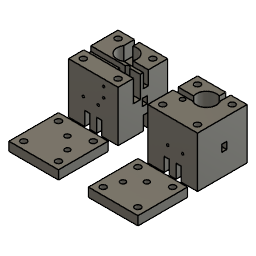
midrail support (Autodesk Fusion 360 design; units mm, degrees)
Autodesk Fusion 360 part; units mm, degrees
note: some values were not read from the file. Chosen so that the rebuilt part matches the saved one: which face or edge a step refers to. Set by a fixed rule: which sketch regions a step uses.
sketch "Sketch1" plane through (0, 0, 0) normal (0, 1, 0) x (1, 0, 0)
  line L0 (25, -25) -> (-25, -25)
  line L1 (-25, -25) -> (-25, 25)
  line L2 (-25, 25) -> (25, 25)
  line L3 (25, 25) -> (25, -25)
  line L4 (25, -25) -> (-25, 25) construction
  line L5 (-25, -25) -> (25, 25) construction
  line L6 (17.5, -17.5) -> (-17.5, -17.5)
  line L7 (-17.5, -17.5) -> (-17.5, 17.5)
  line L8 (-17.5, 17.5) -> (17.5, 17.5)
  line L9 (17.5, 17.5) -> (17.5, -17.5)
  line L10 (17.5, -17.5) -> (-17.5, 17.5) construction
  line L11 (-17.5, -17.5) -> (17.5, 17.5) construction
  circle A0 centre (-17.5, 17.5) radius 1.95
  circle A1 centre (17.5, 17.5) radius 1.95
  circle A2 centre (17.5, -17.5) radius 1.95
  circle A3 centre (-17.5, -17.5) radius 1.95
  line L12 (25, 0) -> (25, 3.5)
  line L13 (-25, 3.5) -> (-25, 0)
  line L14 (25, 0) -> (25, -1.5)
  circle A4 centre (-17.5, 17.5) radius 3
  circle A5 centre (17.5, 17.5) radius 3
  circle A6 centre (17.5, -17.5) radius 3
  circle A7 centre (-17.5, -17.5) radius 3
  line L15 (-25, 2.5) -> (-25, -2.5)
  line L16 (25, -2.5) -> (25, 2.5)
  line L17 (25, 2.5) -> (-25, -2.5) construction
  line L18 (-25, 2.5) -> (25, -2.5) construction
  line L19 (-14.5, -17.5) -> (-13, -17.5)
  line L20 (-13, 17.5) -> (-14.5, 17.5)
  line L21 (-13, -17.5) -> (-8, -17.5)
  line L22 (-8, -25) -> (-13, -25)
  line L23 (-8, -25) -> (-13, -25)
  line L24 (-13, 25) -> (-8, 25)
  line L25 (-10.5, 25) -> (1.5, 25)
  line L26 (1.5, -25) -> (-10.5, -25)
  line L27 (1.5, -25) -> (-1, -25)
  line L28 (1.5, -25) -> (4, -25)
  line L29 (6, -25) -> (-6, -25)
  line L30 (-6, -25) -> (-6, 25)
  line L31 (-6, 25) -> (6, 25)
  line L32 (6, 25) -> (6, -25)
  line L33 (6, -25) -> (-6, 25) construction
  line L34 (-6, -25) -> (6, 25) construction
  line L35 (8.5, -25) -> (3.5, -25)
  line L36 (3.5, -25) -> (3.5, 25)
  line L37 (3.5, 25) -> (8.5, 25)
  line L38 (8.5, 25) -> (8.5, -25)
  line L39 (8.5, -25) -> (3.5, 25) construction
  line L40 (3.5, -25) -> (8.5, 25) construction
  line L41 (-3.5, -25) -> (-8.5, -25)
  line L42 (-8.5, -25) -> (-8.5, 25)
  line L43 (-8.5, 25) -> (-3.5, 25)
  line L44 (-3.5, 25) -> (-3.5, -25)
  line L45 (-3.5, -25) -> (-8.5, 25) construction
  line L46 (-8.5, -25) -> (-3.5, 25) construction
  line L47 (25, 0) -> (-25, 0)
  line L48 (-25, 0) -> (-25, 3)
  line L49 (-25, 3) -> (25, 3)
  line L50 (25, 3) -> (25, 0)
  line L51 (25, 0.5) -> (-25, 0.5)
  line L52 (-25, 0.5) -> (-25, 5.5)
  line L53 (-25, 5.5) -> (25, 5.5)
  line L54 (25, 5.5) -> (25, 0.5)
  line L55 (25, 0.5) -> (-25, 5.5) construction
  line L56 (-25, 0.5) -> (25, 5.5) construction
  line L57 (6, 3) -> (12, 3)
  line L58 (12, 3) -> (12, -3)
  line L59 (12, -3) -> (6, -3)
  line L60 (6, -3) -> (6, 3)
  circle A8 centre (12, -3) radius 10
  line L61 (-6, 3) -> (0, 3)
  line L62 (0, 3) -> (0, 9)
  line L63 (0, 9) -> (-6, 9)
  line L64 (-6, 9) -> (-6, 3)
  circle A9 centre (0, 9) radius 10
  circle A10 centre (12, -3) radius 2.4
  circle A11 centre (0, 9) radius 2.4
  line L65 (25, 3) -> (-25, 3)
  line L66 (-25, 3) -> (-25, -0.5)
  line L67 (-25, -0.5) -> (25, -0.5)
  line L68 (25, -0.5) -> (25, 3)
  line L69 (25, 3) -> (-25, 3)
  line L70 (-25, 3) -> (-25, 4.5)
  line L71 (-25, 4.5) -> (25, 4.5)
  line L72 (25, 4.5) -> (25, 3)
  line L73 (25, -57) -> (-25, -57)
  line L74 (-25, -85) -> (-25, -35)
  line L75 (6, -57) -> (12, -57)
  line L76 (12, -63) -> (6, -63)
  line L77 (-6, -85) -> (-6, -35)
  line L78 (-8.5, -85) -> (-8.5, -35)
  line L79 (17.5, -42.5) -> (17.5, -77.5)
  line L80 (-25, -59.5) -> (-25, -54.5)
  line L81 (1.5, -85) -> (4, -85)
  circle A12 centre (-17.5, -77.5) radius 2.1
  line L82 (-25, -57.5) -> (-25, -62.5)
  line L83 (-25, -60) -> (-25, -57)
  circle A13 centre (17.5, -42.5) radius 2.1
  circle A14 centre (17.5, -77.5) radius 3
  line L84 (-8.5, -85) -> (-3.5, -35) construction
  line L85 (-3.5, -85) -> (-8.5, -35) construction
  line L86 (-25, -57) -> (-25, -55.5)
  line L87 (25, -57) -> (-25, -57)
  line L88 (-17.5, -77.5) -> (17.5, -42.5) construction
  line L89 (-25, -85) -> (25, -35) construction
  circle A15 centre (12, -63) radius 10
  line L90 (-25, -56.5) -> (-25, -60)
  line L91 (-6, -35) -> (6, -35)
  line L92 (6, -85) -> (-6, -35) construction
  circle A16 centre (0, -51) radius 10
  line L93 (25, -60) -> (-25, -60)
  line L94 (25, -59.5) -> (-25, -54.5) construction
  line L95 (-25, -60.5) -> (25, -60.5)
  line L96 (17.5, -77.5) -> (-17.5, -42.5) construction
  line L97 (17.5, -77.5) -> (-17.5, -77.5)
  line L98 (-25, -57) -> (-25, -60.5)
  line L99 (6, -85) -> (-6, -85)
  line L100 (-6, -85) -> (6, -35) construction
  line L101 (-6, -57) -> (0, -57)
  line L102 (-17.5, -77.5) -> (-17.5, -42.5)
  line L103 (-13, -77.5) -> (-8, -77.5)
  line L104 (25, -60.5) -> (25, -57)
  circle A17 centre (17.5, -77.5) radius 2.1
  line L105 (8.5, -35) -> (8.5, -85)
  line L106 (-8, -85) -> (-13, -85)
  line L107 (25, -54.5) -> (25, -59.5)
  line L108 (3.5, -85) -> (8.5, -35) construction
  line L109 (-3.5, -35) -> (-3.5, -85)
  line L110 (1.5, -85) -> (-10.5, -85)
  circle A18 centre (-17.5, -42.5) radius 2.1
  line L111 (25, -57) -> (25, -60)
  line L112 (3.5, -35) -> (8.5, -35)
  line L113 (0, -51) -> (-6, -51)
  line L114 (1.5, -85) -> (-1, -85)
  line L115 (-13, -42.5) -> (-14.5, -42.5)
  line L116 (-3.5, -85) -> (-8.5, -85)
  line L117 (-25, -55.5) -> (25, -55.5)
  line L118 (-17.5, -42.5) -> (17.5, -42.5)
  line L119 (25, -59.5) -> (-25, -59.5)
  line L120 (-25, -35) -> (25, -35)
  line L121 (-25, -57) -> (25, -57)
  line L122 (25, -85) -> (-25, -85)
  line L123 (-25, -59.5) -> (25, -54.5) construction
  circle A19 centre (-17.5, -77.5) radius 3
  circle A20 centre (-17.5, -42.5) radius 3
  line L124 (-25, -54.5) -> (25, -54.5)
  line L125 (25, -57.5) -> (-25, -62.5) construction
  circle A21 centre (12, -63) radius 2.6
  line L126 (6, -63) -> (6, -57)
  line L127 (-6, -51) -> (-6, -57)
  line L128 (-8, -85) -> (-13, -85)
  line L129 (0, -57) -> (0, -51)
  line L130 (-14.5, -77.5) -> (-13, -77.5)
  line L131 (-13, -35) -> (-8, -35)
  line L132 (-10.5, -35) -> (1.5, -35)
  line L133 (8.5, -85) -> (3.5, -35) construction
  circle A22 centre (17.5, -42.5) radius 3
  line L134 (25, -60) -> (25, -56.5)
  line L135 (25, -35) -> (25, -85)
  line L136 (25, -55.5) -> (25, -57)
  line L137 (-8.5, -35) -> (-3.5, -35)
  line L138 (3.5, -85) -> (3.5, -35)
  line L139 (12, -57) -> (12, -63)
  line L140 (25, -62.5) -> (25, -57.5)
  line L141 (6, -35) -> (6, -85)
  line L142 (8.5, -85) -> (3.5, -85)
  line L143 (25, -60) -> (25, -61.5)
  line L144 (25, -85) -> (-25, -35) construction
  line L145 (-25, -57.5) -> (25, -62.5) construction
  circle A23 centre (0, -51) radius 2.6
  point P0 (6, 0)
  point P1 (-6, 0)
  point P2 (0, 3)
  point P3 (0, -57)
  point P4 (0, -60)
  point P5 (0, -60)
  point P6 (-6, -60)
  point P7 (6, -60)
  dimension "d1" = 50
  dimension "d2" = 50
  dimension "d3" = 35
  dimension "d4" = 35
  dimension "d5" = 3.9
  dimension "d6" = 3.9
  dimension "d7" = 3.9
  dimension "d8" = 3.9
  dimension "d11" = 6
  dimension "d12" = 6
  dimension "d13" = 6
  dimension "d14" = 6
  dimension "d15" = 50
  dimension "d135" = 12
  dimension "d136" = 5
  dimension "d137" = 5
  dimension "d138" = 3
  dimension "d139" = 5
  dimension "d140" = 6
  dimension "d141" = 6
  dimension "d142" = 20
  dimension "d143" = 6
  dimension "d144" = 6
  dimension "d145" = 20
  dimension "d146" = 4.8
  dimension "d147" = 4.8
  dimension "d148" = 50
  dimension "d149" = 3.5
  dimension "d150" = 50
  dimension "d151" = 1.5
  dimension "d152" = 50
  dimension "d153" = 50
  dimension "d154" = 35
  dimension "d155" = 35
  dimension "d156" = 4.2
  dimension "d157" = 4.2
  dimension "d158" = 4.2
  dimension "d159" = 4.2
  dimension "d160" = 6
  dimension "d161" = 6
  dimension "d162" = 6
  dimension "d163" = 6
  dimension "d164" = 50
  dimension "d165" = 12
  dimension "d166" = 5
  dimension "d167" = 5
  dimension "d168" = 3
  dimension "d169" = 5
  dimension "d170" = 6
  dimension "d171" = 6
  dimension "d172" = 20
  dimension "d173" = 6
  dimension "d174" = 6
  dimension "d175" = 20
  dimension "d176" = 5.2
  dimension "d177" = 5.2
  dimension "d178" = 50
  dimension "d179" = 3.5
  dimension "d180" = 50
  dimension "d181" = 1.5
  constraint horizontal L0
  constraint perpendicular L0 L1
  constraint parallel L0 L2
  constraint parallel L1 L3
  constraint horizontal L6
  constraint perpendicular L6 L7
  constraint parallel L6 L8
  constraint parallel L7 L9
  constraint coincident L7.end L8.start
  constraint coincident L8.end L9.start
  constraint coincident L6.start L9.end
  constraint coincident L6.end L7.start
  constraint vertical L12
  constraint vertical L13
  constraint midpoint L1 L13.end
  constraint vertical L14
  constraint concentric A0 A4
  constraint concentric A2 A6
  constraint parallel L15 L16
  constraint horizontal L19
  constraint horizontal L20
  constraint coincident L8 L20.start
  constraint coincident A7 L19.start
  constraint coincident L6 L19.start
  constraint horizontal L21
  constraint horizontal L22
  constraint horizontal L23
  constraint horizontal L24
  constraint coincident L2 L24.start
  constraint horizontal L25
  constraint horizontal L26
  constraint coincident L0 L26.start
  constraint midpoint L24 L25.start
  constraint horizontal L27
  constraint horizontal L28
  constraint horizontal L29
  constraint perpendicular L29 L30
  constraint parallel L29 L31
  constraint parallel L30 L32
  constraint coincident L33 origin
  constraint coincident L34 origin
  constraint horizontal L35
  constraint perpendicular L35 L36
  constraint parallel L35 L37
  constraint parallel L36 L38
  constraint coincident L39 P0
  constraint coincident L40 P0
  constraint midpoint L32 P0
  constraint horizontal L41
  constraint perpendicular L41 L42
  constraint parallel L41 L43
  constraint parallel L42 L44
  constraint coincident L45 P1
  constraint coincident L46 P1
  constraint coincident L26 L41.start
  constraint midpoint L30 P1
  constraint horizontal L47
  constraint vertical L48
  constraint horizontal L49
  constraint vertical L50
  constraint horizontal L51
  constraint perpendicular L51 L52
  constraint parallel L51 L53
  constraint parallel L52 L54
  constraint coincident L55 P2
  constraint coincident L56 P2
  constraint midpoint L49 P2
  constraint horizontal L57
  constraint vertical L58
  constraint horizontal L59
  constraint vertical L60
  constraint coincident L32 L57.start
  constraint coincident L49 L57.start
  constraint coincident L58.end L59.start
  constraint horizontal L61
  constraint vertical L62
  constraint horizontal L63
  constraint vertical L64
  constraint coincident L30 L61.start
  constraint coincident L49 L61.start
  constraint coincident L62.end L63.start
  constraint horizontal L65
  constraint vertical L66
  constraint horizontal L67
  constraint vertical L68
  constraint horizontal L69
  constraint vertical L70
  constraint horizontal L71
  constraint vertical L72
  constraint horizontal L122
  constraint perpendicular L74 L122
  constraint parallel L120 L122
  constraint parallel L74 L135
  constraint horizontal L97
  constraint perpendicular L97 L102
  constraint parallel L97 L118
  constraint parallel L79 L102
  constraint coincident L96.end L102.end
  constraint coincident L79.start A13.centre
  constraint coincident L79.end A14.centre
  constraint coincident A12.centre L88.start
  constraint vertical L134
  constraint vertical L90
  constraint midpoint L83.start L74
  constraint vertical L143
  constraint concentric A18 A20
  constraint concentric A14 A17
  constraint parallel L82 L140
  constraint horizontal L130
  constraint horizontal L115
  constraint coincident L115.start L118
  constraint coincident L130.start A19
  constraint coincident L130.start L97
  constraint horizontal L103
  constraint horizontal L106
  constraint horizontal L128
  constraint horizontal L131
  constraint coincident L131.start L120
  constraint horizontal L132
  constraint horizontal L110
  constraint coincident L81.start L122
  constraint midpoint L132.start L131
  constraint horizontal L114
  constraint horizontal L81
  constraint horizontal L99
  constraint perpendicular L77 L99
  constraint parallel L91 L99
  constraint parallel L77 L141
  constraint coincident P5 L92
  constraint coincident P5 L100
  constraint coincident P5 P4
  constraint horizontal L142
  constraint perpendicular L138 L142
  constraint parallel L112 L142
  constraint parallel L105 L138
  constraint coincident P7 L133
  constraint coincident P7 L108
  constraint midpoint P7 L141
  constraint horizontal L116
  constraint perpendicular L78 L116
  constraint parallel L116 L137
  constraint parallel L78 L109
  constraint coincident P6 L85
  constraint coincident P6 L84
  constraint coincident L85.start L110
  constraint midpoint P6 L77
  constraint horizontal L93
  constraint vertical L83
  constraint horizontal L121
  constraint vertical L111
  constraint horizontal L119
  constraint perpendicular L80 L119
  constraint parallel L119 L124
  constraint parallel L80 L107
  constraint coincident P3 L94
  constraint coincident P3 L123
  constraint midpoint P3 L121
  constraint horizontal L75
  constraint vertical L139
  constraint horizontal L76
  constraint vertical L126
  constraint coincident L75.start L141
  constraint coincident L75.start L121
  constraint coincident L76.start A15.centre
  constraint horizontal L101
  constraint vertical L129
  constraint horizontal L113
  constraint vertical L127
  constraint coincident L101.start L77
  constraint coincident L101.start L121
  constraint coincident A16.centre L113.start
  constraint horizontal L87
  constraint vertical L98
  constraint horizontal L95
  constraint vertical L104
  constraint horizontal L73
  constraint vertical L86
  constraint horizontal L117
  constraint vertical L136
  measures "d1" distance of L1.end L2.end
  measures "d2" distance of L0.end L1.end
  measures "d3" distance of L7.end L8.end
  measures "d4" distance of L6.end L7.end
  measures "d5" diameter of A0
  measures "d6" diameter of A1
  measures "d7" diameter of A2
  measures "d8" diameter of A3
  measures "d11" diameter of A4
  measures "d12" diameter of A5
  measures "d13" diameter of A6
  measures "d14" diameter of A7
  measures "d15" distance of L15.end L16.start
  measures "d135" distance of L30.end L31.end
  measures "d136" distance of L36.end L37.end
  measures "d137" distance of L42.end L43.end
  measures "d138" distance of L12.start L49.end
  measures "d139" distance of L51.end L52.end
  measures "d140" distance of L57.start L57.end
  measures "d141" distance of L57.start L59.end
  measures "d142" diameter of A8
  measures "d143" distance of L61.start P2
  measures "d144" distance of L61.start L63.end
  measures "d145" diameter of A9
  measures "d146" diameter of A10
  measures "d147" diameter of A11
  measures "d148" distance of L49.end L48.end
  measures "d149" distance of L49.end L67.end
  measures "d150" distance of L49.end L48.end
  measures "d151" distance of L49.end L71.end
  measures "d152" distance of L89.end L74.end
  measures "d153" distance of L74.start L74.end
  measures "d154" distance of L96.end L79.start
  measures "d155" distance of L96.end A12.centre
  measures "d156" diameter of A18
  measures "d157" diameter of A13
  measures "d158" diameter of A17
  measures "d159" diameter of A12
  measures "d160" diameter of A20
  measures "d161" diameter of A22
  measures "d162" diameter of A14
  measures "d163" diameter of A19
  measures "d164" distance of L82.end L140.start
  measures "d165" distance of L77.end L91.end
  measures "d166" distance of L112.start L105.start
  measures "d167" distance of L78.end L84.end
  measures "d168" distance of L93.start L73.start
  measures "d169" distance of L80.start L80.end
  measures "d170" distance of L75.start L75.end
  measures "d171" distance of L75.start L76.end
  measures "d172" diameter of A15
  measures "d173" distance of P3 L101.start
  measures "d174" distance of L101.start L113.end
  measures "d175" diameter of A16
  measures "d176" diameter of A21
  measures "d177" diameter of A23
  measures "d178" distance of L73.start L73.end
  measures "d179" distance of L73.start L95.end
  measures "d180" distance of L73.start L73.end
  measures "d181" distance of L73.start L117.end
extrude "Extrude1" add sketch "Sketch1" along normal blind 53 contours L0 L3 L6 L9 L14 A6 L16 L38 A8 L67 | L0 L6 L32 L35 L38 | L0 L6 L28 L29 L32 L35 L36 | L6 L9 A6 L38 A8 | L6 L32 L38 A8 | L6 L32 L36 A8 | L6 L9 A2 A6 | L6 L9 A2 A6 | L32 L38 L59 A8 | L9 L38 L58 L59 A8 A10 L67 | L3 L14 L16 L47 A8 L67 L68 | L0 L6 L26 L27 L28 L29 L36 L44 | L6 L36 L44 A8 A9 L67 | L32 L36 L60 A8 L67 | L6 L9 A2 | L6 L9 A2 | L32 L38 L59 L60 L67 | L38 L58 L59 A10 L67 | L9 A8 L67 | L3 L12 L16 L47 L50 L51 A8 L68 | L9 L47 A8 L67 | L0 L6 L26 L29 L30 L41 L44 | L6 L30 L44 L67 | L36 A8 A9 L67 | L32 L38 L47 L60 L67 | L38 L47 L58 L67 | L58 L59 A10 | L58 L59 A10 | L9 L47 L58 L67 | L3 L12 L16 L49 L50 L51 L54 A8 L65 L68 L69 | L9 L47 L51 A8 | L0 L6 L21 L22 L23 L26 L30 L41 L42 | L6 L21 L30 L42 L67 | L30 L44 L47 A9 L67 | L44 A9 L67 | L36 A9 L67 | L32 L36 L47 L60 A9 L67 | A8 A9 L67 | A8 A9 L67 | L32 L38 L47 L51 L60 | L38 L47 L51 L58 | L9 L47 L51 L58 | L9 L49 L51 A8 L65 L69 | L30 L42 L47 L67 | L44 L47 A9 | L44 L47 A8 A9 L67 | L36 L47 A8 A9 L67 | L36 L47 A9 | L32 L47 L51 L60 A9 | L32 L38 L49 L51 L57 L60 A9 L65 L69 | L38 L49 L51 L57 L58 L65 L69 | L9 L49 L51 L58 L65 L69 | L3 L12 L49 L54 A8 L65 L69 L71 L72 | L9 L49 A8 L65 L69 L71 | L0 L1 L6 L7 A7 L15 L19 L21 L22 L23 L26 L42 L67 | L6 L7 A7 L19 L21 L42 L67 | L30 L42 L47 L51 | L30 L47 L51 A9 | L7 L42 L47 L67 | L44 L47 L51 A9 | L44 L47 L51 A8 | L36 L47 L51 A8 | L36 L47 L51 A9 | L32 L51 L60 A9 | L38 L49 L57 A9 L65 L69 | L9 L38 L49 L57 A9 L65 L69 L71 | L9 A8 L71 | L3 L9 L53 L54 A8 L71 | L30 L42 L49 L51 A9 L65 L69 | L30 L51 A9 | L7 L42 L47 L51 | L1 L7 L15 L47 L66 L67 | L30 L44 L49 L51 L61 A9 L65 L69 | L36 L44 L49 L51 A8 L61 L65 L69 | L36 L51 A8 | L32 L36 L49 L51 L60 A8 A9 L65 L69 | L32 L49 L57 L60 A9 L65 L69 | L32 L38 L49 L57 A9 L65 L69 L71 | L38 A9 L71 | L9 L53 A8 A9 L71 | L9 L53 A8 | L6 L7 A3 A7 | L6 L7 A3 A7 | L30 L49 A9 L65 L69 | L7 L42 L49 L51 L65 L69 | L1 L7 L13 L15 L47 L48 L51 L66 | L30 L44 L49 L61 L64 L65 L69 L71 | L44 L49 L61 L62 L65 L69 L71 | L36 L49 A8 L65 L69 | L32 L49 A8 L65 L69 L71 | L32 L38 L53 A8 L71 | L38 L53 A9 L71 | L2 L3 L8 L9 A5 L38 L53 | L8 L9 A5 L38 L53 A8 A9 | L53 A8 A9 | L6 L7 A3 | L6 L7 A3 | L30 L42 L49 L64 A9 L65 L69 L71 | L42 L49 A9 L65 L69 | L7 L42 L49 A9 L65 L69 L71 | L1 L7 L13 L15 L48 L49 L51 L52 L65 L66 L69 | L30 L44 L53 L64 L71 | L44 L53 L62 L71 | L36 L49 L62 L65 L69 L71 | L36 L49 A8 L65 L69 L71 | L32 A8 L71 | L38 L53 A8 | L38 L53 A8 A9 | L8 L9 A1 A5 | L8 L9 A1 A5 | L38 A8 A9 | L30 L42 L53 L64 L71 | L42 A9 L71 | L1 L7 L13 L49 L52 L65 L69 L70 L71 | L30 L44 L53 L63 L64 | L44 L53 L62 L63 A11 | L36 L53 L62 L71 | L32 L36 L53 A8 L71 | L32 L53 A8 | L32 L38 L53 A8 A9 | L2 L8 L32 L37 L38 | L8 L9 A1 | L8 L9 A1 | L30 L42 L53 L64 A9 | L42 L53 A9 L71 | L7 L53 A9 L71 | L1 L7 L52 L53 L71 | L8 L30 L44 L63 A9 | L8 L36 L44 L53 L62 L63 A11 | L8 L32 L36 L53 A9 | L8 L32 L38 A9 | L2 L8 L31 L32 L36 L37 A9 | L42 L53 A9 | L7 L8 A4 L20 L42 L53 A9 | L1 L2 L7 L8 A4 L20 L24 L25 L42 L53 | L8 L36 L44 A9 | L8 L44 A9 | L62 L63 A11 | L62 L63 A11 | L8 L36 A9 | L8 L32 A9 | L2 L25 L31 L36 L44 A9 | L8 L30 L42 A9 | L8 L30 A9 | L7 L8 A0 A4 | L7 L8 A0 A4 | L2 L8 L25 L30 L31 L43 L44 A9 | L2 L8 L24 L25 L30 L42 L43 | L7 L8 A0 | L7 L8 A0 makes body 1
extrude "Extrude2" cut sketch "Sketch1" along normal blind 53 contours L6 L9 A2 A6 | L6 L9 A2 A6 | L6 L9 A2 | L6 L9 A2 | L58 L59 A10 | L58 L59 A10 | L6 L7 A3 A7 | L6 L7 A3 A7 | L6 L7 A3 | L6 L7 A3 | L8 L9 A1 A5 | L8 L9 A1 A5 | L8 L9 A1 | L8 L9 A1 | L62 L63 A11 | L62 L63 A11 | L7 L8 A0 A4 | L7 L8 A0 A4 | L7 L8 A0 | L7 L8 A0 bodies 1
extrude "Extrude3" cut sketch "Sketch1" along normal blind 23 and the other way blind -30 contours L3 L14 L16 L47 A8 L67 L68 | L3 L12 L16 L47 L50 L51 A8 L68 | L9 L47 A8 L67 | L32 L38 L47 L60 L67 | L38 L47 L58 L67 | L9 L47 L58 L67 | L3 L12 L16 L49 L50 L51 L54 A8 L65 L68 L69 | L9 L47 L51 A8 | L30 L44 L47 A9 L67 | L44 A9 L67 | L36 A9 L67 | L32 L36 L47 L60 A9 L67 | L32 L38 L47 L51 L60 | L38 L47 L51 L58 | L9 L47 L51 L58 | L9 L49 L51 A8 L65 L69 | L30 L42 L47 L67 | L44 L47 A9 | L44 L47 A8 A9 L67 | L36 L47 A8 A9 L67 | L36 L47 A9 | L32 L47 L51 L60 A9 | L32 L38 L49 L51 L57 L60 A9 L65 L69 | L38 L49 L51 L57 L58 L65 L69 | L9 L49 L51 L58 L65 L69 | L3 L12 L49 L54 A8 L65 L69 L71 L72 | L9 L49 A8 L65 L69 L71 | L30 L42 L47 L51 | L30 L47 L51 A9 | L7 L42 L47 L67 | L44 L47 L51 A9 | L44 L47 L51 A8 | L36 L47 L51 A8 | L36 L47 L51 A9 | L32 L51 L60 A9 | L38 L49 L57 A9 L65 L69 | L9 L38 L49 L57 A9 L65 L69 L71 | L30 L42 L49 L51 A9 L65 L69 | L30 L51 A9 | L7 L42 L47 L51 | L1 L7 L15 L47 L66 L67 | L30 L44 L49 L51 L61 A9 L65 L69 | L36 L44 L49 L51 A8 L61 L65 L69 | L36 L51 A8 | L32 L36 L49 L51 L60 A8 A9 L65 L69 | L32 L49 L57 L60 A9 L65 L69 | L32 L38 L49 L57 A9 L65 L69 L71 | L38 A9 L71 | L30 L49 A9 L65 L69 | L7 L42 L49 L51 L65 L69 | L1 L7 L13 L15 L47 L48 L51 L66 | L30 L44 L49 L61 L64 L65 L69 L71 | L44 L49 L61 L62 L65 L69 L71 | L36 L49 A8 L65 L69 | L32 L49 A8 L65 L69 L71 | L30 L42 L49 L64 A9 L65 L69 L71 | L42 L49 A9 L65 L69 | L7 L42 L49 A9 L65 L69 L71 | L1 L7 L13 L15 L48 L49 L51 L52 L65 L66 L69 | L36 L49 L62 L65 L69 L71 | L36 L49 A8 L65 L69 L71 | L42 A9 L71 | L1 L7 L13 L49 L52 L65 L69 L70 L71 bodies 1
extrude "Extrude4" cut sketch "Sketch1" along normal blind 15 contours L0 L6 L32 L35 L38 | L0 L6 L28 L29 L32 L35 L36 | L6 L32 L38 A8 | L6 L32 L36 A8 | L32 L38 L59 A8 | L9 L38 L58 L59 A8 A10 L67 | L32 L36 L60 A8 L67 | L32 L38 L59 L60 L67 | L38 L58 L59 A10 L67 | L9 A8 L67 | L9 L47 A8 L67 | L0 L6 L26 L29 L30 L41 L44 | L6 L30 L44 L67 | L36 A8 A9 L67 | L32 L38 L47 L60 L67 | L38 L47 L58 L67 | L9 L47 L58 L67 | L3 L12 L16 L49 L50 L51 L54 A8 L65 L68 L69 | L9 L47 L51 A8 | L0 L6 L21 L22 L23 L26 L30 L41 L42 | L6 L21 L30 L42 L67 | L30 L44 L47 A9 L67 | L36 A9 L67 | L32 L36 L47 L60 A9 L67 | A8 A9 L67 | L32 L38 L47 L51 L60 | L38 L47 L51 L58 | L9 L47 L51 L58 | L9 L49 L51 A8 L65 L69 | L30 L42 L47 L67 | L44 L47 A9 | L36 L47 A8 A9 L67 | L36 L47 A9 | L32 L47 L51 L60 A9 | L32 L38 L49 L51 L57 L60 A9 L65 L69 | L38 L49 L51 L57 L58 L65 L69 | L9 L49 L51 L58 L65 L69 | L3 L12 L49 L54 A8 L65 L69 L71 L72 | L9 L49 A8 L65 L69 L71 | L30 L42 L47 L51 | L30 L47 L51 A9 | L44 L47 L51 A9 | L36 L47 L51 A8 | L36 L47 L51 A9 | L32 L51 L60 A9 | L38 L49 L57 A9 L65 L69 | L9 L38 L49 L57 A9 L65 L69 L71 | L9 A8 L71 | L3 L9 L53 L54 A8 L71 | L30 L42 L49 L51 A9 L65 L69 | L30 L51 A9 | L30 L44 L49 L51 L61 A9 L65 L69 | L36 L51 A8 | L32 L36 L49 L51 L60 A8 A9 L65 L69 | L32 L49 L57 L60 A9 L65 L69 | L32 L38 L49 L57 A9 L65 L69 L71 | L38 A9 L71 | L9 L53 A8 A9 L71 | L30 L49 A9 L65 L69 | L30 L44 L49 L61 L64 L65 L69 L71 | L32 L49 A8 L65 L69 L71 | L32 L38 L53 A8 L71 | L38 L53 A9 L71 | L53 A8 A9 | L30 L42 L49 L64 A9 L65 L69 L71 | L42 L49 A9 L65 L69 | L30 L44 L53 L64 L71 | L32 A8 L71 | L38 L53 A8 | L38 L53 A8 A9 | L30 L42 L53 L64 L71 | L30 L44 L53 L63 L64 | L30 L42 L53 L64 A9 | L8 L30 L44 L63 A9 | L8 L44 A9 | L8 L30 L42 A9 | L8 L30 A9 | L2 L8 L25 L30 L31 L43 L44 A9 | L2 L8 L24 L25 L30 L42 L43 picked at (2.5677, -0.5863) bodies 1
extrude "Extrude5" cut sketch "Sketch1" along normal blind 53 and the other way blind -38 contours L3 L12 L16 L49 L50 L51 L54 A8 L65 L68 L69 | A8 A9 L67 | A8 A9 L67 | L9 L49 L51 A8 L65 L69 | L44 L47 A9 | L44 L47 A8 A9 L67 | L36 L47 A8 A9 L67 | L36 L47 A9 | L32 L38 L49 L51 L57 L60 A9 L65 L69 | L38 L49 L51 L57 L58 L65 L69 | L9 L49 L51 L58 L65 L69 | L3 L12 L49 L54 A8 L65 L69 L71 L72 | L9 L49 A8 L65 L69 L71 | L44 L47 L51 A9 | L44 L47 L51 A8 | L36 L47 L51 A8 | L36 L47 L51 A9 | L32 L51 L60 A9 | L38 L49 L57 A9 L65 L69 | L9 L38 L49 L57 A9 L65 L69 L71 | L9 A8 L71 | L3 L9 L53 L54 A8 L71 | L30 L44 L49 L51 L61 A9 L65 L69 | L36 L44 L49 L51 A8 L61 L65 L69 | L36 L51 A8 | L32 L36 L49 L51 L60 A8 A9 L65 L69 | L32 L49 L57 L60 A9 L65 L69 | L32 L38 L49 L57 A9 L65 L69 L71 | L38 A9 L71 | L9 L53 A8 A9 L71 | L9 L53 A8 | L30 L49 A9 L65 L69 | L30 L44 L49 L61 L64 L65 L69 L71 | L44 L49 L61 L62 L65 L69 L71 | L36 L49 A8 L65 L69 | L32 L49 A8 L65 L69 L71 | L32 L38 L53 A8 L71 | L38 L53 A9 L71 | L30 L42 L49 L64 A9 L65 L69 L71 | L30 L44 L53 L64 L71 | L44 L53 L62 L71 | L36 L49 L62 L65 L69 L71 | L36 L49 A8 L65 L69 L71 | L32 A8 L71 | L38 L53 A8 | L38 L53 A8 A9 | L38 A8 A9 | L30 L42 L53 L64 L71 | L42 A9 L71 | L30 L44 L53 L63 L64 | L44 L53 L62 L63 A11 | L36 L53 L62 L71 | L32 L36 L53 A8 L71 | L32 L53 A8 | L32 L38 L53 A8 A9 | L30 L42 L53 L64 A9 | L42 L53 A9 L71 | L8 L30 L44 L63 A9 | L8 L36 L44 L53 L62 L63 A11 | L8 L32 L36 L53 A9 | L42 L53 A9 | L8 L36 L44 A9 | L8 L44 A9 | L8 L36 A9 | L8 L30 L42 A9 | L8 L30 A9 | L2 L8 L25 L30 L31 L43 L44 A9 | L2 L8 L24 L25 L30 L42 L43 bodies 1
extrude "Extrude6" add sketch "Sketch1" along normal blind 10 separate body contours L73 L87 A15 L104 L107 L111 L119 L121 L134 L135 L140 | L73 L87 A15 L107 L117 L121 L134 L135 L136 | L73 L79 L87 A15 L119 L121 | L73 L79 L87 A15 L117 L121 | L73 L79 L87 L119 L121 L139 | L73 L75 L79 L87 A16 L105 L117 L121 | A15 L93 L104 L111 L119 L134 L135 L140 | L79 A15 L93 L119 | L79 A15 L117 | L79 A15 L107 L117 L124 L135 | L73 L75 L87 L105 L119 L121 L139 | L79 A15 A16 L117 L124 | L79 L93 L119 L139 | A15 L93 L95 L104 L135 L140 L143 | L79 A15 L93 L95 | L79 A15 L124 | L79 L105 L118 L120 L124 A22 L135 | L73 L75 L87 A16 L105 L119 L121 L126 L141 | L73 L75 L87 A16 L105 L121 | L93 L105 L119 L139 | A16 L105 L117 L124 | A16 L105 L117 | L79 L93 L95 A21 L139 | L79 A14 A15 L95 L97 L105 L122 L135 L140 L143 | L79 A15 L95 | L79 A15 A16 L105 L118 L124 A22 | A15 A16 L124 | L73 L75 L87 A16 L121 L126 L141 | L73 L75 L87 A16 L105 L117 L121 L141 | L93 L105 L119 L126 L141 | L93 L95 L105 A21 L139 | A15 A16 L105 L124 | A15 L105 L117 L124 L141 | L76 L79 A15 L95 L105 A21 | L79 A13 L118 A22 | L79 A13 L118 A22 | A15 A16 L105 | L105 L112 L118 L120 L141 | L73 L87 A15 A16 L119 L121 L126 L138 L141 | L73 L87 A15 L117 L121 L141 | A16 L119 L126 L141 | L93 L95 L105 L126 L141 | A16 L93 L119 L126 L141 | L95 A21 L139 | L95 A21 L139 | A15 L105 L124 | A15 L117 L141 | L79 A14 A15 L97 L105 | L76 L95 A21 L139 | L79 A13 L118 | L79 A13 L118 | A15 A16 L105 L124 L141 | A16 L105 L118 L141 | L91 A16 L112 L118 L120 L138 L141 | L73 L87 A15 L121 L138 | L73 L87 A15 L117 L121 L138 | A16 L93 L119 L138 | A16 L93 L95 L126 L138 L141 | L76 L95 L105 L126 L141 | L76 L95 L105 A21 | L76 L95 A21 L139 | A15 L124 L141 | A15 L117 L124 L138 L141 | L79 A14 L97 A17 | L79 A14 L97 A17 | A15 L97 L105 L141 | L76 A15 L105 L141 | A16 L118 L141 | L91 A16 L109 L120 L132 L138 | L73 L87 A15 L101 L109 L119 L121 L138 | L73 L87 L117 L121 L129 L138 | A15 L119 L138 | A16 L93 L138 | A15 L93 L119 L138 | A15 L95 L126 L138 L141 | A16 L118 L124 L138 L141 | L117 L124 L129 L138 | L79 L97 A17 | L79 L97 A17 | A15 L97 L138 L141 | L97 L105 L122 L141 L142 | A16 L118 L138 | A16 L109 L118 L138 | L73 L87 L101 L109 L117 L121 L129 | A15 L93 L109 L119 | A16 L95 L138 | A15 A16 L93 L95 L138 | A15 A16 L95 L138 | L109 L113 L118 L124 L129 L138 A23 | L109 L117 L124 L129 | A15 A16 L95 L97 L109 L138 | L81 L97 L99 L122 L138 L141 L142 | L77 L91 A16 L109 L118 L120 L132 L137 | A16 L109 L118 | L73 L77 L87 A16 L101 L109 L119 L121 | L73 L77 L87 L101 L109 L117 L121 L127 | A15 A16 L93 L95 L109 | A16 L93 L109 L119 | A15 A16 L95 | L109 L113 L124 L129 A23 | L77 L109 L117 L124 L127 | A15 A16 L95 | L81 L97 L99 L109 L110 L114 L122 L138 | L77 A16 L109 L113 L118 | L77 L78 L118 L120 L131 L132 L137 | L77 A16 L118 | L73 L77 L87 A16 L121 | L73 L77 L78 L87 A16 L117 L121 L127 | A16 L93 L109 | L77 A16 L119 | L77 A16 L93 L119 | L77 L109 L113 L124 L127 | L113 L129 A23 | L113 L129 A23 | L77 L78 L117 L124 L127 | A16 L95 L109 | L77 L97 L99 L109 L110 L116 L122 | L77 L95 L97 L109 | L77 L78 A16 L118 | L77 L78 A16 L124 L127 | L73 L77 L78 L87 A16 L119 L121 | L73 L78 L87 A16 L121 | L77 A16 L93 L95 L109 | L77 L78 L93 L119 | L78 A16 L117 L124 | L78 A16 L117 | L77 L78 L95 L97 L103 | L77 L78 L97 L103 L106 L110 L116 L122 L128 | L74 L78 L102 L115 L118 L120 A20 L124 L131 L132 | L78 A16 L102 L115 L118 A20 L124 | L78 A16 L124 | L73 L78 L87 L102 L119 L121 | L73 L78 L87 A16 L102 L117 L121 | L77 L78 L93 L95 | L78 L93 L102 L119 | A16 L102 L117 L124 | L73 L74 L80 L82 L83 L87 L90 L98 L102 L119 L121 | L73 L74 L80 L86 L87 L90 L102 L117 L121 | L78 L93 L95 L102 | L74 L82 L83 L90 L93 L98 L102 L119 | L74 L80 L102 L117 L124 | L78 L95 L97 L102 L103 A19 L130 | L74 L78 L82 L95 L97 L102 L103 L106 L110 L122 A19 L128 L130 | L102 A18 L118 A20 | L102 A18 L118 A20 | L74 L82 L93 L95 L98 L102 | L102 A18 L118 | L102 A18 L118 | A12 L97 L102 A19 | A12 L97 L102 A19 | A12 L97 L102 | A12 L97 L102 makes body 2
extrude "Extrude7" cut sketch "Sketch1" along normal blind 10 contours L79 A13 L118 A22 | L79 A13 L118 A22 | L95 A21 L139 | L95 A21 L139 | L76 L95 A21 L139 | L79 A13 L118 | L79 A13 L118 | L76 L95 A21 L139 | L79 A14 L97 A17 | L79 A14 L97 A17 | L79 L97 A17 | L79 L97 A17 | L113 L129 A23 | L113 L129 A23 | L102 A18 L118 A20 | L102 A18 L118 A20 | L102 A18 L118 | L102 A18 L118 | A12 L97 L102 A19 | A12 L97 L102 A19 | A12 L97 L102 | A12 L97 L102 bodies 2
copy_body "CopyPasteBodies1" bodies 1 makes body 3
move_body "Move1" bodies 3 to x (-1, 0, 0) y (0, -1, 0) z (0, 0, 1) at (60, 53, 0)
copy_body "CopyPasteBodies2" bodies 2 makes body 4
move_body "Move2" bodies 4 to x (-1, 0, 0) y (0, -1, 0) z (0, 0, 1) at (60, 10, 0)
extrude "Extrude8" cut 5 faces at (17.4167, 53, -9.4302) (56.0299, 53, -18.0604) (70.599, 53, 5.3994) (49.0323, 53, 18.5725) (-0.1361, 53, 11.6991) along direction (0, -1, 0) blind 1 on bodies 1 3 bodies 1 3
extrude "Extrude9" cut 5 faces at (60.1361, 0, 11.6991) (42.5833, 0, -9.4302) (3.9701, 0, -18.0604) (10.9677, 0, 18.5725) (-10.599, 0, 5.3994) along direction (0, 1, 0) blind 1 on bodies 1 3 bodies 1 3
move_body "Move3" bodies 2 4 to x (1, 0, 0) y (0, 1, 0) z (0, 0, 1) at (0, 1, 0)
extrude "Extrude10" cut 2 faces at (71.9377, 11, 57.4882) (-11.9377, 11, 57.4882) along direction (0, -1, 0) blind 1 on bodies 2 4 bodies 2 4
move_body "Move4" bodies 3 4 to x (1, 0, 0) y (0, 1, 0) z (0, 0, 1) at (595, 0, 0)
sketch "Sketch2" plane through (0, 0, 25) normal (0, 0, 1) x (1, 0, 0)
  line L0 (8.5, 1) -> (25, 1)
  line L1 (25, 1) -> (25, 52)
  line L2 (25, 52) -> (-25, 52)
  line L3 (-25, 52) -> (-25, 1)
  line L4 (-25, 1) -> (-8.5, 1)
  line L5 (-8.5, 1) -> (-8.5, 15)
  line L6 (-8.5, 15) -> (-3.5, 15)
  line L7 (-3.5, 15) -> (-3.5, 1)
  line L8 (-3.5, 1) -> (3.5, 1)
  line L9 (3.5, 1) -> (3.5, 15)
  line L10 (3.5, 15) -> (8.5, 15)
  line L11 (8.5, 15) -> (8.5, 1)
  line L12 (25, 52) -> (-25, 52)
  line L13 (-25, 52) -> (-25, 30)
  line L14 (-25, 30) -> (25, 30)
  line L15 (25, 30) -> (25, 52)
  line L16 (-25, 30) -> (680, 30)
  line L17 (680, 30) -> (680, 23)
  line L18 (680, 23) -> (-25, 23)
  line L19 (-25, 23) -> (-25, 30)
  line L20 (680, 26.5) -> (665, 26.5)
  line L21 (665, 26.5) -> (650, 26.5)
  line L22 (650, 26.5) -> (635, 26.5)
  line L23 (635, 26.5) -> (620, 26.5)
  line L24 (-25, 26.5) -> (-10, 26.5)
  line L25 (-10, 26.5) -> (5, 26.5)
  line L26 (5, 26.5) -> (20, 26.5)
  circle A0 centre (665, 26.5) radius 1.15
  circle A1 centre (650, 26.5) radius 1.15
  circle A2 centre (635, 26.5) radius 1.15
  circle A3 centre (20, 26.5) radius 1.15
  circle A4 centre (5, 26.5) radius 1.15
  circle A5 centre (-10, 26.5) radius 1.15
  dimension "d188" = 22
  dimension "d189" = 705
  dimension "d190" = 7
  dimension "d191" = 15
  dimension "d192" = 15
  dimension "d193" = 15
  dimension "d194" = 15
  dimension "d195" = 15
  dimension "d196" = 15
  dimension "d197" = 15
  dimension "d198" = 2.3
  dimension "d199" = 2.3
  dimension "d200" = 2.3
  dimension "d201" = 2.3
  dimension "d202" = 2.3
  dimension "d203" = 2.3
  constraint horizontal L12
  constraint vertical L13
  constraint horizontal L14
  constraint vertical L15
  constraint coincident L1.end L2.start
  constraint horizontal L16
  constraint vertical L17
  constraint horizontal L18
  constraint vertical L19
  constraint midpoint L17 L20.start
  constraint perpendicular L17 L20
  constraint parallel L20 L21
  constraint parallel L21 L22
  constraint parallel L16 L23
  constraint midpoint L19 L24.start
  constraint perpendicular L19 L24
  constraint parallel L24 L25
  constraint parallel L25 L26
  constraint coincident L20.end L21.start
  constraint coincident L21.end L22.start
  constraint coincident L22.end L23.start
  constraint coincident L26.end A3.centre
  constraint coincident L25.end L26.start
  constraint coincident L24.end L25.start
  measures "d188" distance of L1.end L14.end
  measures "d189" distance of L13.end L16.end
  measures "d190" distance of L13.end L18.end
  measures "d191" distance of L20.start L20.end
  measures "d192" distance of L20.end L21.end
  measures "d193" distance of L21.end L22.end
  measures "d194" distance of L22.end L23.end
  measures "d195" distance of L24.start L24.end
  measures "d196" distance of L24.end L25.end
  measures "d197" distance of L25.end L26.end
  measures "d198" diameter of A0
  measures "d199" diameter of A1
  measures "d200" diameter of A2
  measures "d201" diameter of A3
  measures "d202" diameter of A4
  measures "d203" diameter of A5
extrude "Extrude11" cut sketch "Sketch2" against normal blind 50 contours L20 L21 A0 | L20 L21 A0 | L21 L22 A1 | L21 L22 A1 | L24 L25 A5 | L24 L25 A5 | L25 L26 A4 | L25 L26 A4 bodies 1 3
move_body "Move5" bodies 3 4 to x (1, 0, 0) y (0, 1, 0) z (0, 0, 1) at (-590, 0, 0)
move_body "Move6" bodies 3 4 to x (1, 0, 0) y (0, 1, 0) z (0, 0, 1) at (170, 0, 0)
mirror "Mirror1" about plane through (25, 0, 2.5) normal (1, 0, 0) of bodies 1 2 makes body 5 at (75, 25.3333, 16.8333) makes body 6 at (61.9377, 10, 57.4882)
move_body "Move8" bodies 5 6 to x (1, 0, 0) y (0, 1, 0) z (0, 0, 1) at (30, 0, 0)
sketch "Sketch3" plane through (25, 0, 0) normal (1, 0, 0) x (0, 0, -1)
  line L0 (4.5, 23) -> (-0.5, 23)
  line L1 (-0.5, 23) -> (-0.5, 30)
  line L2 (-0.5, 30) -> (4.5, 30)
  line L3 (4.5, 30) -> (4.5, 23)
  line L4 (-25, 1) -> (0.5, 1)
  line L5 (0.5, 1) -> (0.5, 15)
  line L6 (0.5, 15) -> (5.5, 15)
  line L7 (5.5, 15) -> (5.5, 1)
  line L8 (5.5, 1) -> (25, 1)
  line L9 (25, 1) -> (25, 52)
  line L10 (25, 52) -> (5.5, 52)
  line L11 (5.5, 52) -> (5.5, 38)
  line L12 (5.5, 38) -> (0.5, 38)
  line L13 (0.5, 38) -> (0.5, 52)
  line L14 (0.5, 52) -> (-25, 52)
  line L15 (-25, 52) -> (-25, 1)
  line L16 (-0.5, 30) -> (-2.5, 30)
  line L17 (-2.5, 30) -> (-9.5, 30)
  line L18 (-9.5, 30) -> (-9.5, 52)
  line L19 (-9.5, 52) -> (-2.5, 52)
  line L20 (-2.5, 52) -> (-2.5, 30)
  line L21 (-9.5, 52) -> (-2.5, 52)
  line L22 (-2.5, 52) -> (-2.5, 32)
  line L23 (-2.5, 32) -> (-9.5, 32)
  line L24 (-9.5, 32) -> (-9.5, 52)
  line L25 (-9.5, 52) -> (-2.5, 52)
  line L26 (-2.5, 52) -> (-2.5, 47)
  line L27 (-2.5, 47) -> (-9.5, 47)
  line L28 (-9.5, 47) -> (-9.5, 52)
  dimension "d208" = 2
  dimension "d209" = 7
  dimension "d210" = 22
  dimension "d211" = 7
  dimension "d212" = 20
  dimension "d217" = 7
  dimension "d218" = 5
  constraint coincident L1.end L2.start
  constraint perpendicular L1 L16
  constraint horizontal L17
  constraint vertical L18
  constraint horizontal L19
  constraint vertical L20
  constraint horizontal L21
  constraint vertical L22
  constraint horizontal L23
  constraint vertical L24
  constraint horizontal L25
  constraint vertical L26
  constraint horizontal L27
  constraint vertical L28
  measures "d208" distance of L1.end L16.end
  measures "d209" distance of L16.end L17.end
  measures "d210" distance of L16.end L19.end
  measures "d211" distance of L18.end L19.end
  measures "d212" distance of L18.end L23.end
  measures "d217" distance of L18.end L19.end
  measures "d218" distance of L18.end L27.end
extrude "Extrude12" cut sketch "Sketch3" against normal blind 21 contours L14 L18 L19 L20 L21 L22 L24 L25 L26 L27 L28 | L18 L20 L22 L23 L24 L27 bodies 1
extrude "Extrude13" cut sketch "Sketch3" against normal blind 21 contours L17 L18 L20 L23 bodies 1
extrude "Extrude14" cut sketch "Sketch3" against normal blind 50 contours L14 L18 L19 L20 L21 L22 L24 L25 L26 L27 L28 bodies 1
sketch "Sketch4" plane through (0, 0, 9.5) normal (0, 0, -1) x (-1, 0, 0)
  line L0 (-25, 52) -> (-25, 30)
  line L1 (-25, 30) -> (-4, 30)
  line L2 (-4, 30) -> (-4, 47)
  line L3 (-4, 47) -> (25, 47)
  line L4 (25, 47) -> (25, 52)
  line L5 (25, 52) -> (-25, 52)
  line L6 (-4, 52) -> (-10.5, 52)
  line L7 (-10.5, 52) -> (-10.5, 45.5)
  line L8 (-10.5, 45.5) -> (-4, 45.5)
  line L9 (-4, 45.5) -> (-4, 52)
  line L10 (-10.5, 45.5) -> (-10.5, 35.5)
  circle A0 centre (-10.5, 45.5) radius 1.1
  circle A1 centre (-10.5, 35.5) radius 1.1
  dimension "d221" = 6.5
  dimension "d222" = 6.5
  dimension "d223" = 10
  dimension "d224" = 2.2
  dimension "d225" = 2.2
  constraint horizontal L6
  constraint vertical L7
  constraint horizontal L8
  constraint vertical L9
  constraint coincident L5 L6.start
  constraint vertical L10
  constraint coincident L7.end L8.start
  constraint coincident L10.end A1.centre
  measures "d221" distance of L6.start L6.end
  measures "d222" distance of L6.start L8.end
  measures "d223" distance of L7.end L10.end
  measures "d224" diameter of A0
  measures "d225" diameter of A1
extrude "Extrude15" cut sketch "Sketch4" against normal blind 15.5 contours L7 L8 A0 | L7 L10 A0 | L8 L10 A0 | A1 bodies 1
hidden bodies 3 4
equation "d2 = d1"
equation "d4 = d3"
equation "d6 = d5"
equation "d7 = d5"
equation "d8 = d5"
equation "d12 = d11"
equation "d13 = d11"
equation "d14 = d11"
equation "d42 = -53.00 mm + 15 mm"
equation "d153 = d1"
equation "d155 = d3"
equation "d161 = d11"
equation "d162 = d11"
equation "d163 = d11"
equation "d189 = ( 15 * 47 ) * 1 mm"
